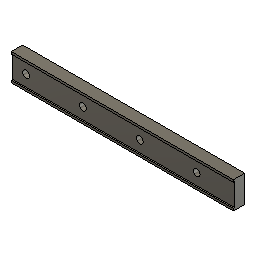
Rear+Axle+Support+Spacer+v3 (Autodesk Fusion 360 archive; units mm, degrees)
design "Rear Axle Support Spacer v3" references "haas mini mill-edu"
Autodesk Fusion 360 part; units mm, degrees
sketch "Sketch1" plane through (0, 0, 0) normal (0, 1, 0) x (1, 0, 0)
  line L0 (0, 0) -> (48.26, 0)
  line L1 (48.26, 0) -> (48.26, -24.257)
  line L2 (48.26, -24.257) -> (0, -24.257)
  line L3 (0, -24.257) -> (0, 0)
  line L4 (0, -1.397) -> (48.26, -1.397)
  line L5 (48.26, -1.397) -> (48.26, -22.86)
  line L6 (48.26, -22.86) -> (0, -22.86)
  line L7 (0, -22.86) -> (0, -1.397)
  line L8 (0, -12.1285) -> (48.26, -12.1285) construction
  circle A0 centre (12.827, -12.1285) radius 3.175
  line L9 (0, -12.1285) -> (12.827, -12.1285)
  line L10 (51.562, -1.397) -> (99.822, -1.397)
  line L11 (51.562, 0) -> (99.822, 0)
  line L12 (99.822, -1.397) -> (99.822, -22.86)
  line L13 (51.562, -12.1285) -> (99.822, -12.1285) construction
  line L14 (99.822, -24.257) -> (51.562, -24.257)
  circle A1 centre (64.389, -12.1285) radius 3.175
  line L15 (99.822, -22.86) -> (51.562, -22.86)
  line L16 (51.562, -24.257) -> (51.562, 0)
  line L17 (51.562, -22.86) -> (51.562, -1.397)
  line L18 (99.822, 0) -> (99.822, -24.257)
  line L19 (51.562, -12.1285) -> (64.389, -12.1285)
  line L20 (-3.302, 0) -> (206.248, 0)
  line L21 (103.124, -1.397) -> (151.384, -1.397)
  line L22 (151.384, -1.397) -> (151.384, -22.86)
  line L23 (151.384, -24.257) -> (103.124, -24.257)
  line L24 (103.124, -22.86) -> (103.124, -1.397)
  line L25 (103.124, -12.1285) -> (115.951, -12.1285)
  circle A2 centre (115.951, -12.1285) radius 3.175
  line L26 (151.384, -22.86) -> (103.124, -22.86)
  line L27 (103.124, -12.1285) -> (151.384, -12.1285) construction
  line L28 (151.384, 0) -> (151.384, -24.257)
  line L29 (103.124, 0) -> (151.384, 0)
  line L30 (103.124, -24.257) -> (103.124, 0)
  line L31 (154.686, -1.397) -> (202.946, -1.397)
  line L32 (202.946, -1.397) -> (202.946, -22.86)
  line L33 (202.946, -24.257) -> (154.686, -24.257)
  line L34 (154.686, -22.86) -> (154.686, -1.397)
  line L35 (154.686, -12.1285) -> (167.513, -12.1285)
  circle A3 centre (167.513, -12.1285) radius 3.175
  line L36 (202.946, -22.86) -> (154.686, -22.86)
  line L37 (154.686, -12.1285) -> (202.946, -12.1285) construction
  line L38 (202.946, 0) -> (202.946, -24.257)
  line L39 (154.686, 0) -> (202.946, 0)
  line L40 (154.686, -24.257) -> (154.686, 0)
  line L41 (-3.302, 0) -> (206.248, 0)
  line L42 (206.248, 0) -> (206.248, -24.257)
  line L43 (206.248, -24.257) -> (-3.302, -24.257)
  line L44 (-3.302, -24.257) -> (-3.302, 0)
  point P0 (51.562, 0)
  point P1 (103.124, 0)
  point P2 (154.686, 0)
  dimension "d1" = 48.26
  dimension "d2" = 24.257
  dimension "d3" = 21.463
  dimension "d4" = 6.35
  dimension "d6" = 12.827
  dimension "d11" = 48.26
  dimension "d12" = 24.257
  dimension "d13" = 21.463
  dimension "d14" = 6.35
  dimension "d15" = 12.827
  dimension "d17" = 48.26
  dimension "d18" = 24.257
  dimension "d19" = 21.463
  dimension "d20" = 6.35
  dimension "d21" = 12.827
  dimension "d22" = 48.26
  dimension "d23" = 24.257
  dimension "d24" = 21.463
  dimension "d25" = 6.35
  dimension "d26" = 12.827
  dimension "d27" = 3.302
  dimension "d28" = 3.302
  dimension "d29" = 3.302
  dimension "d30" = 3.302
  dimension "d31" = 3.302
  dimension "d32" = 209.55
  dimension "d33" = 24.257
  constraint horizontal L0
  constraint vertical L1
  constraint horizontal L2
  constraint vertical L3
  constraint horizontal L4
  constraint vertical L5
  constraint horizontal L6
  constraint vertical L7
  constraint coincident L1 L5.end
  constraint coincident L3 L4.start
  constraint midpoint L3 L8.start
  constraint midpoint L1 L8.end
  constraint symmetric L4 L6 L8
  constraint coincident L8 A0.centre
  constraint perpendicular L7 L9
  constraint coincident A0.centre L9.end
  constraint horizontal L11
  constraint vertical L18
  constraint horizontal L14
  constraint vertical L16
  constraint coincident P0 L11.start
  constraint horizontal L10
  constraint vertical L12
  constraint horizontal L15
  constraint vertical L17
  constraint coincident L12.end L18
  constraint coincident L10.start L16
  constraint midpoint L13.start L16
  constraint midpoint L13.end L18
  constraint symmetric L10 L13 L15
  constraint coincident A1.centre L13
  constraint perpendicular L17 L19
  constraint coincident A1.centre L19.end
  constraint perpendicular L12 L20
  constraint horizontal L29
  constraint vertical L28
  constraint horizontal L23
  constraint vertical L30
  constraint coincident P1 L29.start
  constraint horizontal L21
  constraint vertical L22
  constraint horizontal L26
  constraint vertical L24
  constraint coincident L22.end L28
  constraint coincident L21.start L30
  constraint midpoint L25.start L30
  constraint midpoint L27.end L28
  constraint symmetric L21 L26 L27
  constraint coincident L25.end L27
  constraint perpendicular L24 L25
  constraint coincident L25.end A2.centre
  constraint horizontal L39
  constraint vertical L38
  constraint horizontal L33
  constraint vertical L40
  constraint coincident P2 L39.start
  constraint horizontal L31
  constraint vertical L32
  constraint horizontal L36
  constraint vertical L34
  constraint coincident L32.end L38
  constraint coincident L31.start L40
  constraint midpoint L35.start L40
  constraint midpoint L37.end L38
  constraint symmetric L31 L36 L37
  constraint coincident L35.end L37
  constraint perpendicular L34 L35
  constraint coincident L35.end A3.centre
  constraint coincident L0.start L20
  constraint horizontal L41
  constraint vertical L42
  constraint horizontal L43
  constraint vertical L44
  measures "d1" distance of L0.start L0.end
  measures "d2" distance of L0.end L1.end
  measures "d3" distance of L4 L6
  measures "d4" diameter of A0
  measures "d6" distance of L8.start A0.centre
  measures "d11" distance of L11.end P0
  measures "d12" distance of L11.end L14.start
  measures "d13" distance of L10 L15
  measures "d14" diameter of A1
  measures "d15" distance of A1.centre L13.start
  measures "d17" distance of L28.start P1
  measures "d18" distance of L23.start L28.start
  measures "d19" distance of L21 L26
  measures "d20" diameter of A2
  measures "d21" distance of L25.end L25.start
  measures "d22" distance of L38.start P2
  measures "d23" distance of L33.start L38.start
  measures "d24" distance of L31 L36
  measures "d25" diameter of A3
  measures "d26" distance of L35.end L35.start
  measures "d27" distance of L28 L34
  measures "d28" distance of L18 L30
  measures "d29" distance of L5 L16
  measures "d30" distance of L20.end L38
  measures "d31" distance of L0.start L20.start
  measures "d32" distance of L20.start L20.end
  measures "d33" distance of L20.start L43.end
extrude "Extrude1" [suppressed]
extrude "Extrude2" [suppressed]
extrude "Extrude3" [suppressed]
sketch "Sketch2" plane through (0, 0, 0) normal (0, 1, 0) x (1, 0, 0)
  line L0 (0, 0) -> (208.28, 0)
  line L1 (208.28, 0) -> (208.28, 25.3746)
  line L2 (208.28, 25.3746) -> (0, 25.3746)
  line L3 (0, 25.3746) -> (0, 0)
  line L4 (208.28, 12.6873) -> (0, 12.6873) construction
  circle A0 centre (12.573, 12.6873) radius 3.175
  line L5 (48.26, 25.3746) -> (48.26, 0) construction
  line L6 (53.34, 25.3746) -> (53.34, 0) construction
  line L7 (101.6, 25.3746) -> (101.6, 0) construction
  line L8 (106.68, 25.3746) -> (106.68, 0) construction
  line L9 (154.94, 25.3746) -> (154.94, 0) construction
  line L10 (160.02, 25.3746) -> (160.02, 0) construction
  circle A1 centre (65.913, 12.6873) radius 3.175
  circle A2 centre (119.253, 12.6873) radius 3.175
  circle A3 centre (172.593, 12.6873) radius 3.175
  dimension "d36" = 208.28
  dimension "d37" = 25.3746
  dimension "d38" = 48.26
  dimension "d39" = 5.08
  dimension "d42" = 53.34
  dimension "d43" = 0
  dimension "d44" = 6.35
  dimension "d52" = 12.573
  dimension "d55" = 53.34
  dimension "d56" = 0
  constraint horizontal L0
  constraint vertical L1
  constraint horizontal L2
  constraint vertical L3
  constraint coincident L0.start L3.end
  constraint midpoint L1 L4.start
  constraint midpoint L3 L4.end
  constraint coincident L4 A0.centre
  constraint coincident L2 L5.start
  constraint coincident L0 L5.end
  constraint perpendicular L0 L5
  constraint coincident L2 L6.start
  constraint coincident L0 L6.end
  constraint perpendicular L0 L6
  measures "d36" distance of L0.start L0.end
  measures "d37" distance of L0.start L2.end
  measures "d38" distance of L3 L5
  measures "d39" distance of L5 L6
  measures "d44" diameter of A0
  measures "d52" distance of L3 A0.centre
extrude "Extrude4" add sketch "Sketch2" along normal blind 9.398
sketch "Sketch3" plane through (0, 9.398, 0) normal (0, 1, 0) x (-1, 0, 0)
  circle A0 centre (-65.913, -12.6873) radius 3.175
  circle A1 centre (-12.573, -12.6873) radius 3.175
  circle A2 centre (-172.593, -12.6873) radius 3.175
  circle A3 centre (-119.253, -12.6873) radius 3.175
  line L0 (0, -25.3746) -> (0, 0)
  line L1 (0, 0) -> (-208.28, 0)
  line L2 (-208.28, 0) -> (-208.28, -25.3746)
  line L3 (-208.28, -25.3746) -> (0, -25.3746)
  line L4 (0, -25.3746) -> (-208.28, -25.3746)
  line L5 (-208.28, -25.3746) -> (-208.28, -23.2918)
  line L6 (-208.28, -23.2918) -> (0, -23.2918)
  line L7 (0, -23.2918) -> (0, -25.3746)
  line L8 (0, 0) -> (-208.28, 0)
  line L9 (-208.28, 0) -> (-208.28, -2.0828)
  line L10 (-208.28, -2.0828) -> (0, -2.0828)
  line L11 (0, -2.0828) -> (0, 0)
  dimension "d60" = 21.209
  constraint horizontal L4
  constraint vertical L5
  constraint horizontal L6
  constraint vertical L7
  constraint coincident L2 L5.end
  constraint coincident L0.start L3.end
  constraint horizontal L8
  constraint vertical L9
  constraint horizontal L10
  constraint vertical L11
  constraint coincident L2 L9.end
  constraint coincident L0.end L1.start
  constraint equal L7 L11
  measures "d60" distance of L6 L10
extrude "Extrude5" add sketch "Sketch3" along normal blind 1.27 contours L0 L2 L3 L4 L5 L6 L7 | L0 L1 L2 L8 L9 L10 L11
move_body "Move1" bodies 1 to x (1, 0, 0) y (0, 0, 1) z (0, -1, 0) at (0, -25.3746, -25.3746)
equation "d6 = 0.38 in + 0.125 in"
equation "d15 = 0.38 in + 0.125 in"
equation "d21 = 0.38 in + 0.125 in"
equation "d26 = 0.38 in + 0.125 in"
equation "d36 = TotalLength"
equation "d37 = TotalWidth"
equation "d38 = SpacerLength"
equation "d39 = SpacerGap"
equation "d42 = SpacerGap + SpacerLength"
equation "d44 = HoleDiam"
equation "SpacerLength = 1.9 in"
equation "SpacerGap = ( TotalLength - 4 * SpacerLength ) / 3"
equation "HoleDiam = 0.25 in"
equation "TotalWidth = 0.999 in"
equation "FlangeWidth = 0.835 in"
equation "TotalLength = 8.2 in"
equation "HoleDistance = 0.37 in + HoleDiam / 2"
equation "d52 = HoleDistance"
equation "d55 = SpacerGap + SpacerLength"
equation "SpacerHeight = 0.37 in"
equation "d58 = SpacerHeight"
equation "d60 = FlangeWidth"
